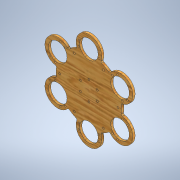
# Autodesk Inventor part: GenevaHolder
Saved by Autodesk Inventor 2020.2 (Build 242310000, 310)
## iProperties
Created: 2019-11-06
Part Number: GenevaHolder
Material: Plywood, Finish
Document SubType Name: Modeling
Designer: Paul Lefeuvre
Density: 0.552 g/cm^3
Appearance: Plywood - New
Author: Paul Lefeuvre
Autodesk Inventor part; units mm, degrees
ref_plane "YZ Plane" through (0, 0, 0) normal (1, 0, 0) x (0, 1, 0)
ref_plane "XZ Plane" through (0, 0, 0) normal (0, 1, 0) x (-1, 0, 0)
ref_plane "XY Plane" through (0, 0, 0) normal (0, 0, 1) x (1, 0, 0)
sketch "Sketch1" plane through (0, 0, 0) normal (0, 0, 1) x (1, 0, 0)
  circle A0 centre (0, 0) radius 186.2 construction
  line L0 (0, 0) -> (0, 152.9684) construction
  circle A1 centre (0, 0) radius 100 construction
  circle A2 centre (0, 148.1) radius 38.1
  circle A3 centre (0, 148.1) radius 37.5 construction
  arc A4 (-52.8521, 124.2242) -> (-81.1553, 107.8834) centre (0, 0) ccw
  arc A5 (-134.0074, 16.3409) -> (-134.0074, -16.3409) centre (0, 0) ccw
  arc A6 (-81.1553, -107.8834) -> (-52.8521, -124.2242) centre (0, 0) ccw
  arc A7 (52.8521, -124.2242) -> (81.1553, -107.8834) centre (0, 0) ccw
  arc A8 (134.0074, -16.3409) -> (134.0074, 16.3409) centre (0, 0) ccw
  arc A9 (81.1553, 107.8834) -> (52.8521, 124.2242) centre (0, 0) ccw
  arc A10 (50.0927, 130.4839) -> (-50.0927, 130.4839) centre (0, 148.1) ccw
  arc A11 (-52.8521, 124.2242) -> (-50.0927, 130.4839) centre (-54.8096, 128.8251) ccw
  arc A12 (50.0927, 130.4839) -> (52.8521, 124.2242) centre (54.8096, 128.8251) ccw
  arc A13 (-87.956, 108.6235) -> (-138.0487, 21.8604) centre (-128.2584, 74.05) ccw
  circle A14 centre (-128.2584, 74.05) radius 38.1
  arc A15 (-87.956, 108.6235) -> (-81.1553, 107.8834) centre (-84.161, 111.879) ccw
  arc A16 (-134.0074, 16.3409) -> (-138.0487, 21.8604) centre (-138.9706, 16.9461) ccw
  arc A17 (-138.0487, -21.8604) -> (-87.956, -108.6235) centre (-128.2584, -74.05) ccw
  circle A18 centre (-128.2584, -74.05) radius 38.1
  arc A19 (-138.0487, -21.8604) -> (-134.0074, -16.3409) centre (-138.9706, -16.9461) ccw
  arc A20 (-81.1553, -107.8834) -> (-87.956, -108.6235) centre (-84.161, -111.879) ccw
  arc A21 (-50.0927, -130.4839) -> (50.0927, -130.4839) centre (0, -148.1) ccw
  circle A22 centre (0, -148.1) radius 38.1
  arc A23 (-50.0927, -130.4839) -> (-52.8521, -124.2242) centre (-54.8096, -128.8251) ccw
  arc A24 (52.8521, -124.2242) -> (50.0927, -130.4839) centre (54.8096, -128.8251) ccw
  arc A25 (87.956, -108.6235) -> (138.0487, -21.8604) centre (128.2584, -74.05) ccw
  circle A26 centre (128.2584, -74.05) radius 38.1
  arc A27 (87.956, -108.6235) -> (81.1553, -107.8834) centre (84.161, -111.879) ccw
  arc A28 (134.0074, -16.3409) -> (138.0487, -21.8604) centre (138.9706, -16.9461) ccw
  arc A29 (138.0487, 21.8604) -> (87.956, 108.6235) centre (128.2584, 74.05) ccw
  circle A30 centre (128.2584, 74.05) radius 38.1
  arc A31 (138.0487, 21.8604) -> (134.0074, 16.3409) centre (138.9706, 16.9461) ccw
  arc A32 (81.1553, 107.8834) -> (87.956, 108.6235) centre (84.161, 111.879) ccw
  circle A33 centre (41.5415, 160.1) radius 3.3
  circle A34 centre (41.5415, 136.1) radius 3.3
  line L1 (0, 148.1) -> (41.5415, 160.1) construction
  line L2 (41.5415, 160.1) -> (41.5415, 136.1) construction
  line L3 (41.5415, 136.1) -> (0, 148.1) construction
  circle A35 centre (-41.5415, 160.1) radius 3.3
  circle A36 centre (-41.5415, 136.1) radius 3.3
  circle A37 centre (-117.8799, 116.026) radius 3.3
  circle A38 centre (-97.0953, 104.026) radius 3.3
  circle A39 centre (-159.4214, 44.074) radius 3.3
  circle A40 centre (-138.6368, 32.074) radius 3.3
  circle A41 centre (-159.4214, -44.074) radius 3.3
  circle A42 centre (-138.6368, -32.074) radius 3.3
  circle A43 centre (-117.8799, -116.026) radius 3.3
  circle A44 centre (-97.0953, -104.026) radius 3.3
  circle A45 centre (-41.5415, -160.1) radius 3.3
  circle A46 centre (-41.5415, -136.1) radius 3.3
  circle A47 centre (41.5415, -160.1) radius 3.3
  circle A48 centre (41.5415, -136.1) radius 3.3
  circle A49 centre (117.8799, -116.026) radius 3.3
  circle A50 centre (97.0953, -104.026) radius 3.3
  circle A51 centre (159.4214, -44.074) radius 3.3
  circle A52 centre (138.6368, -32.074) radius 3.3
  circle A53 centre (159.4214, 44.074) radius 3.3
  circle A54 centre (138.6368, 32.074) radius 3.3
  circle A55 centre (117.8799, 116.026) radius 3.3
  circle A56 centre (97.0953, 104.026) radius 3.3
  circle A57 centre (0, 0) radius 72.5 construction
  line L4 (0, 0) -> (293.3984, 0) construction
  line L5 (0, 0) -> (-240, 0) construction
  circle A58 centre (0, 40) radius 3.9
  circle A59 centre (-34.641, 20) radius 3.9
  circle A60 centre (-34.641, -20) radius 3.9
  circle A61 centre (0, -40) radius 3.9
  circle A62 centre (34.641, -20) radius 3.9
  circle A63 centre (34.641, 20) radius 3.9
  circle A64 centre (-120, 0) radius 3.9
  circle A65 centre (-60, -103.923) radius 3.9
  circle A66 centre (60, -103.923) radius 3.9
  circle A67 centre (120, 0) radius 3.9
  circle A68 centre (60, 103.923) radius 3.9
  circle A69 centre (-60, 103.923) radius 3.9
  point P0 (-34.3824, 131.6848)
  point P1 (-32.4194, 128.0852)
  point P2 (34.2525, 131.4155)
  point P3 (32.4194, 128.0852)
  point P4 (-94.7153, 92.1186)
  point P5 (-127.1347, 35.9666)
  point P6 (-131.2335, 36.0663)
  point P7 (-96.6829, 95.3713)
  point P8 (-127.1347, -35.9666)
  point P9 (-94.7153, -92.1186)
  point P10 (-96.8511, -95.6184)
  point P11 (-130.9354, -36.0442)
  point P12 (-32.4194, -128.0852)
  point P13 (32.4194, -128.0852)
  point P14 (34.3824, -131.6848)
  point P15 (-34.2525, -131.4155)
  point P16 (94.7153, -92.1186)
  point P17 (127.1347, -35.9666)
  point P18 (131.2335, -36.0663)
  point P19 (96.6829, -95.3713)
  point P20 (127.1347, 35.9666)
  point P21 (94.7153, 92.1186)
  point P22 (96.8511, 95.6184)
  point P23 (130.9354, 36.0442)
  dimension "d0" = 372.4
  dimension "d42" = 0.6
  dimension "d43" = 135
  dimension "d44" = 75
  dimension "d45" = 15
  dimension "d48" = 5
  dimension "d51" = 360
  dimension "d53" = 6.6
  dimension "d54" = 6.6
  dimension "d56" = 43.24
  dimension "d57" = 24
  dimension "d58" = 43.24
  dimension "d61" = 360
  dimension "d64" = 200
  dimension "d65" = 145
  dimension "d73" = 7.8
  dimension "d74" = 40
  dimension "d77" = 360
  dimension "d79" = 7.8
  dimension "d80" = 120
  dimension "d83" = 360
  constraints: 72 point on circle, 70 centre point, 12 end point, 7 coincident, 6 equal radius, 5 tangent, 2 horizontal, 2 point on line, 2 symmetric about line, 2 vertical, 1 midpoint, 168 other
  measures "d0" diameter of A0
  measures "d42" radial gap between concentric circles of A2 A3
  measures "d43" radius of A9
  measures "d44" diameter of A3
  measures "d45" radial gap between concentric circles of A2 A10
  measures "d48" radius of A11
  measures "d53" diameter of A33
  measures "d54" diameter of A34
  measures "d56" distance of L1.start L1.end
  measures "d57" distance of L1.end L2.end
  measures "d58" distance of L2.end L3.end
  measures "d64" diameter of A1
  measures "d65" diameter of A57
  measures "d73" diameter of A58
  measures "d74" distance of A58.centre L0.start
  measures "d79" diameter of A64
  measures "d80" distance of point (0, 0) A64.centre
extrude "Extrusion1" add sketch "Sketch1" along normal blind 9
body "Solid1"
